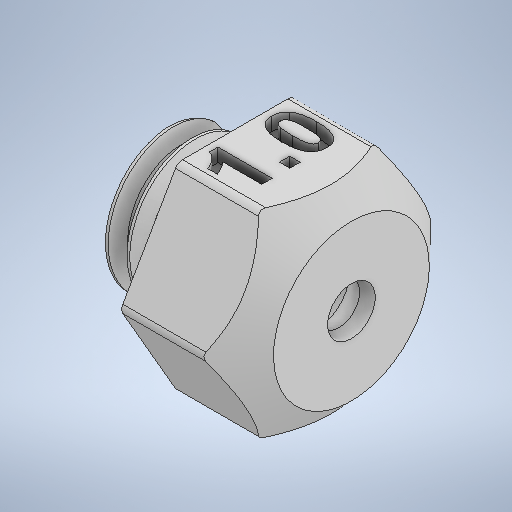
# Autodesk Inventor part: Part1
Saved by Autodesk Inventor 2025.2 (Build 292293000, 293)
## iProperties
Created: 2026-03-09
Part Number: Part1
Material: Generic
Document SubType Name: Modeling
Designer: Simon
Density: 1 g/cm^3
Appearance: Default
Author: Simon
Autodesk Inventor part; units mm, degrees
ref_plane "YZ Plane" through (0, 0, 0) normal (1, 0, 0) x (0, 1, 0)
ref_plane "XZ Plane" through (0, 0, 0) normal (0, 1, 0) x (-1, 0, 0)
ref_plane "XY Plane" through (0, 0, 0) normal (0, 0, 1) x (1, 0, 0)
sketch "Sketch1" plane through (0, 0, 0) normal (0, 0, 1) x (1, 0, 0)
  line L0 (0, 0) -> (0, 1.25)
  line L1 (0, 1.25) -> (50, 1.25)
  line L2 (0, 0) -> (0, 0.7609)
  line L3 (0, 0.7609) -> (50, 0.7609)
  line L4 (0, 0) -> (0, 0.8835)
  line L5 (0, 0.8835) -> (50, 0.8835)
  line L6 (0, 0) -> (0, 2.5)
  line L7 (0, 2.5) -> (2.5, 2.5)
  line L8 (2.5, 2.5) -> (2.5, 1.25)
  line L9 (2.5, 1.25) -> (2.5, 4.25)
  line L10 (2.5, 1.25) -> (6.7109, 1.25) construction
  line L11 (2.5, 4.25) -> (5.5, 4.25)
  line L12 (5.5, 4.25) -> (5.5, 1.25)
  line L13 (5.5, 1.25) -> (6.3472, 0.7609)
  line L14 (5.5, 1.25) -> (9.25, 1.25) construction
  line L15 (6.3472, 0.7609) -> (6.8047, 0.8835)
  line L16 (6.3472, 0.7609) -> (6.8208, 0.7609) construction
  line L17 (6.8047, 0.8835) -> (6.8047, 2.8835)
  line L18 (6.8047, 2.8835) -> (5.5, 4.25)
  line L19 (0, 0) -> (50, 0)
  dimension "d0" = 1.25
  dimension "d1" = 50
  dimension "d2" = 0.7609
  dimension "d3" = 0.8835
  dimension "d4" = 2.5
  dimension "d5" = 2.5
  dimension "d6" = 3
  dimension "d8" = 3
  dimension "d9" = 30
  dimension "d10" = 15
  dimension "d12" = 2
  dimension "d13" = 50
  constraints: 40 end point, 7 perpendicular, 7 point on line, 5 horizontal, 2 vertical, 1 equal length
  measures "d0" distance of L0.start L0.end
  measures "d1" distance of L0.end L1.end
  measures "d2" distance of L0.start L2.end
  measures "d3" distance of L0.start L4.end
  measures "d4" distance of L0.start L6.end
  measures "d5" distance of L6.end L7.end
  measures "d6" distance of L8.end L9.end
  measures "d8" distance of L9.end L11.end
  measures "d9" angle of L13 L14
  measures "d10" angle of L16 L15
  measures "d12" distance of L15.end L17.end
  measures "d13" distance of L0.start L19.end
revolve "Revolution1" add sketch "Sketch1" angle 360 about axis through (0, 0, 0) along (1, 0, 0) contours L13 L5 L15 | L6 L7 L8 L1 | L13 L1 L17 L5 | L8 L9 L11 L12 L1 | L12 L18 L17 L1
sketch "Sketch2" plane through (2.5, 0, 0) normal (-1, 0, 0) x (0, 0, 1)
  circle A0 centre (0, 0) radius 4.25 projected
  line L0 (-4.25, 0) -> (4.25, 0)
  circle A1 centre (0, 0) radius 0.7609 projected
  line L1 (4.25, 0) -> (2.125, -3.6806)
  line L2 (2.125, -3.6806) -> (-2.125, -3.6806)
  line L3 (-2.125, -3.6806) -> (-4.25, 0)
  line L4 (-4.25, 0) -> (-2.125, 3.6806)
  line L5 (-2.125, 3.6806) -> (2.125, 3.6806)
  line L6 (2.125, 3.6806) -> (4.25, 0)
  circle A2 centre (0, 0) radius 1.25
  constraints: 14 end point, 2 coincident, 2 point on circle, 1 centre point, 1 horizontal, 13 other
extrude "Extrusion1" cut sketch "Sketch2" against normal through all contours L6 A0 | A0 L1 | L5 A0 | A0 L2 | L4 A0 | A0 L3
fillet "Fillet1" radius 0.3 6 edges at (4, 3.6806, 2.125) (4, 3.6806, -2.125) (4, 0, -4.25) (4, -3.6806, -2.125) (4, -3.6806, 2.125) (4, 0, 4.25)
sketch "Sketch3" plane through (0, 0, 0) normal (0, 0, 1) x (1, 0, 0)
  line L0 (-0.35, 1.8938) -> (0.45, 1.8938)
  line L1 (-0.35, 1.8938) -> (0.05, 2.5866)
  line L2 (-0.35, 1.8938) -> (0.45, 1.8938) construction
  line L3 (0.05, 2.5866) -> (0.45, 1.8938)
  line L4 (-0.0972, 3.8266) -> (0.7028, 3.8266) construction
  line L5 (0.05, 2.5866) -> (0.05, 1.8938)
  line L6 (0.05, 1.8938) -> (0.05, 2.0671)
  line L7 (0.05, 2.0671) -> (0.45, 2.0671)
  line L8 (0.45, 2.0671) -> (-0.35, 2.0671)
  line L9 (0.05, 2.5866) -> (0.05, 2.5)
  line L10 (0.05, 2.5) -> (0.45, 2.5)
  line L11 (0.45, 2.5) -> (-0.35, 2.5)
  line L12 (-0.35, 1.8938) -> (-1.15, 1.8938)
  line L13 (0.05, 2.5866) -> (-0.75, 2.5866)
  line L14 (-0.75, 2.5866) -> (-1.15, 1.8938)
  line L15 (-0.35, 1.8938) -> (-0.75, 2.5866)
  line L16 (-0.35, 2.0671) -> (-1.15, 2.0671)
  line L17 (-0.35, 2.5) -> (-0.8, 2.5)
  line L18 (-0.75, 2.5866) -> (-0.75, 1.8938)
  line L19 (-0.35, 1.8938) -> (-0.35, 1.9938)
  circle A0 centre (-0.35, 2.0938) radius 0.1
  line L20 (-0.4077, 1.9938) -> (-0.2923, 1.9938)
  line L21 (0, 2.5) -> (2.5, 2.5) projected
  line L22 (0, 2.5) -> (-0.7, 2.5)
  line L23 (-0.7, 2.5) -> (-0.4366, 2.0438)
  line L24 (-0.4366, 2.0438) -> (-0.2634, 2.0438)
  line L25 (-0.2634, 2.0438) -> (0, 2.5)
  circle A1 centre (-0.35, 2.0938) radius 0.1
  point P0 (0, 0)
  point P1 (0, 2.5)
  dimension "d18" = 0.8
  dimension "d19" = 60
  dimension "d20" = 60
  dimension "d21" = 0.1732
  dimension "d22" = 0.0866
  dimension "d23" = 0.8
  dimension "d24" = 0.1
  dimension "d25" = 0.8
  constraints: 50 end point, 13 point on line, 7 horizontal, 4 tangent, 3 midpoint, 2 centre point, 2 equal length, 2 perpendicular, 2 point on circle, 1 coincident, 1 collinear, 1 concentric, 1 parallel, 1 vertical
  measures "d18" distance of L2.start L0.end
  measures "d19" angle of L2 L1
  measures "d20" angle of L3 L4
  measures "d21" distance of L6.start L7.start
  measures "d22" distance of L3.start L10.start
  measures "d23" distance of L2.start L12.end
  measures "d24" distance of L2.start L19.end
  measures "d25" distance between parallel lines of L5 L18
coil "Coil1" sketch "Sketch3" operation cut axis through (-10, 0, 0) along (1, 0, 0) pitch 0.8 turns 4 hand right contours A0 L24 | L24 L15 L16 L8 L1 | A0 L15 L17 L11 L1 | L8 L16 A0
extrude "Extrusion2" add sketch "Sketch2" against normal blind 3 contours L1 L2 L3 L0 A2 | L0 A2 L4 L5 L6
fillet "Fillet2" radius 0.3 6 edges at (4, 3.6806, -2.125) (4, 3.6806, 2.125) (4, 0, 4.25) (4, -3.6806, 2.125) (4, -3.6806, -2.125) (4, 0, -4.25)
sketch "Sketch4" plane through (2.5, 3.6806, 1.9518) normal (0, 1, 0) x (1, 0, 0)
  line L0 (0.2517, -0.0394) -> (0.2517, 3.8177) construction
  line L1 (0.2517, 3.8177) -> (2.7552, 3.8177) construction
  line L2 (2.7552, 3.8177) -> (2.7552, -0.0394) construction
  line L3 (2.7552, -0.0394) -> (0.2517, -0.0394) construction
  line L4 (2.2593, 1.0612) -> (2.2593, 0.677)
  line L5 (2.2593, 0.677) -> (0.8157, 0.677)
  spline S0 degree 2 poles (0.8157, 0.677) (1.0109, 0.4667) (1.1054, 0.1816) knots 0 0 0 1 1 1
  line L6 (1.1054, 0.1816) -> (0.7578, 0.1816)
  spline S1 degree 2 poles (0.7578, 0.1816) (0.709, 0.3325) (0.4346, 0.6846) (0.2517, 0.7502) knots 0 0 0 1 2 2 2
  line L7 (0.2517, 0.7502) -> (0.2517, 1.0612)
  line L8 (0.2517, 1.0612) -> (2.2593, 1.0612)
  line L9 (2.2593, 1.7136) -> (1.8752, 1.7136)
  line L10 (1.8752, 1.7136) -> (1.8752, 2.0978)
  line L11 (1.8752, 2.0978) -> (2.2593, 2.0978)
  line L12 (2.2593, 2.0978) -> (2.2593, 1.7136)
  spline S2 degree 2 poles (0.2517, 3.0566) (0.2517, 3.3478) (0.459, 3.5109) knots 0 0 0 1 1 1
  spline S3 degree 2 poles (0.459, 3.5109) (0.7045, 3.706) (1.2731, 3.706) knots 0 0 0 1 1 1
  spline S4 degree 2 poles (1.2731, 3.706) (1.8401, 3.706) (2.0886, 3.5093) knots 0 0 0 1 1 1
  spline S5 degree 2 poles (2.0886, 3.5093) (2.2929, 3.3478) (2.2929, 3.0566) knots 0 0 0 1 1 1
  spline S6 degree 2 poles (2.2929, 3.0566) (2.2929, 2.7639) (1.8447, 2.4072) (1.2685, 2.4072) knots 0 0 0 1 2 2 2
  spline S7 degree 2 poles (1.2685, 2.4072) (0.7045, 2.4072) (0.456, 2.6038) knots 0 0 0 1 1 1
  spline S8 degree 2 poles (0.456, 2.6038) (0.2517, 2.7654) (0.2517, 3.0566) knots 0 0 0 1 1 1
  spline S9 degree 2 poles (0.5703, 3.0566) (0.5703, 2.9865) (0.6587, 2.8782) (0.7731, 2.8478) knots 0 0 0 1 2 2 2
  spline S10 degree 2 poles (0.7731, 2.8478) (0.9209, 2.8081) (1.2731, 2.8081) knots 0 0 0 1 1 1
  spline S11 degree 2 poles (1.2731, 2.8081) (1.6237, 2.8081) (1.8874, 2.8798) (1.9743, 2.9865) (1.9743, 3.0566) knots 0 0 0 1 2 3 3 3
  spline S12 degree 2 poles (1.9743, 3.0566) (1.9743, 3.1267) (1.8859, 3.2349) (1.7715, 3.2654) knots 0 0 0 1 2 2 2
  spline S13 degree 2 poles (1.7715, 3.2654) (1.6237, 3.3051) (1.2731, 3.3051) knots 0 0 0 1 1 1
  spline S14 degree 2 poles (1.2731, 3.3051) (0.9209, 3.3051) (0.6587, 3.2334) (0.5703, 3.1267) (0.5703, 3.0566) knots 0 0 0 1 2 3 3 3
  point P0 (-2.5, 1.9518)
  constraints: 2 other
extrude "Extrusion3" cut sketch "Sketch4" against normal blind 0.5
body "Solid1"
